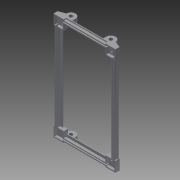
# Autodesk Inventor part: Lid2
Saved by Autodesk Inventor 2015 (Build 190159000, 159)
## iProperties
Created: 2015-03-20
Part Number: Lid2
Material: NylonD2W
Document SubType Name: Modeling
Designer: Akovo_000
Density: 0.93 g/cm^3
Appearance: Nylon 6
Mass: 32.4877 g
Surface Area: 348.455 cm^2
Volume: 34.933 cm^3
Author: Akovo_000
Autodesk Inventor part; units mm, degrees
ref_plane "YZ Plane" through (0, 0, 0) normal (1, 0, 0) x (0, 1, 0)
ref_plane "XZ Plane" through (0, 0, 0) normal (0, 1, 0) x (-1, 0, 0)
ref_plane "Main Work Pane" through (0, 2.75, 7) normal (0, 1, 0) x (-1, 0, 0)
sketch "Panel" plane through (0, 2.75, 7) normal (0, 1, 0) x (-1, 0, 0)
  line L0 (90.0297, -97.7451) -> (-32.1703, -97.7451)
  line L1 (-32.1703, -97.7451) -> (-32.1703, 113.4549)
  line L2 (-32.1703, 113.4549) -> (90.0297, 113.4549)
  line L3 (90.0297, 113.4549) -> (90.0297, -97.7451)
  line L4 (71.9297, 95.3549) -> (88.0297, 95.3549)
  line L5 (88.0297, 95.3549) -> (88.0297, 111.4549)
  line L6 (88.0297, 111.4549) -> (71.9297, 111.4549)
  line L7 (71.9297, 111.4549) -> (71.9297, 95.3549)
  line L8 (69.9297, 113.4549) -> (69.9297, 93.3549)
  line L9 (69.9297, 93.3549) -> (90.0297, 93.3549)
  line L10 (88.0297, -95.7451) -> (71.9297, -95.7451)
  line L11 (71.9297, -95.7451) -> (71.9297, -79.6451)
  line L12 (71.9297, -79.6451) -> (88.0297, -79.6451)
  line L13 (88.0297, -79.6451) -> (88.0297, -95.7451)
  line L14 (90.0297, -77.6451) -> (69.9297, -77.6451)
  line L15 (69.9297, -77.6451) -> (69.9297, -97.7451)
  line L16 (-30.1703, -95.7451) -> (-14.0703, -95.7451)
  line L17 (-14.0703, -95.7451) -> (-14.0703, -79.6451)
  line L18 (-14.0703, -79.6451) -> (-30.1703, -79.6451)
  line L19 (-30.1703, -79.6451) -> (-30.1703, -95.7451)
  line L20 (-12.0703, -97.7451) -> (-12.0703, -77.6451)
  line L21 (-12.0703, -77.6451) -> (-32.1703, -77.6451)
  line L22 (-14.0703, 95.3549) -> (-30.1703, 95.3549)
  line L23 (-30.1703, 95.3549) -> (-30.1703, 111.4549)
  line L24 (-30.1703, 111.4549) -> (-14.0703, 111.4549)
  line L25 (-14.0703, 111.4549) -> (-14.0703, 95.3549)
  line L26 (-12.0703, 113.4549) -> (-12.0703, 93.3549)
  line L27 (-12.0703, 93.3549) -> (-32.1703, 93.3549)
  circle A0 centre (76.9297, 100.3549) radius 2
  circle A1 centre (-19.0703, 100.3549) radius 2
  circle A2 centre (76.9297, -84.6451) radius 2
  circle A3 centre (-19.0703, -84.6451) radius 2
  line L28 (-19.0703, -84.6451) -> (-14.0703, -84.6451) construction
  line L29 (-19.0703, -84.6451) -> (-19.0703, -79.6451) construction
  line L30 (76.9297, -84.6451) -> (71.9297, -84.6451) construction
  line L31 (76.9297, -84.6451) -> (76.9297, -79.6451) construction
  line L32 (76.9297, 100.3549) -> (76.9297, 95.3549) construction
  line L33 (76.9297, 100.3549) -> (71.9297, 100.3549) construction
  line L34 (-19.0703, 100.3549) -> (-14.0703, 100.3549) construction
  line L35 (-19.0703, 100.3549) -> (-19.0703, 95.3549) construction
  line L36 (69.9297, 100.3549) -> (-12.0703, 100.3549)
  line L37 (76.9297, 93.3549) -> (76.9297, -77.6451)
  line L38 (69.9297, -84.6451) -> (-12.0703, -84.6451)
  line L39 (-19.0703, 93.3549) -> (-19.0703, -77.6451)
  dimension "d584" = 2
  dimension "d585" = 2
  dimension "d586" = 2
  dimension "d587" = 2
  dimension "d588" = 16.1
  dimension "d589" = 16.1
  dimension "d592" = 2
  dimension "d593" = 4
  dimension "d597" = 2
  dimension "d648" = 2
  dimension "d661" = 5
  dimension "d670" = 175
  dimension "d671" = 86
  dimension "d682" = 211.2
  dimension "d687" = 122.2
  constraints: 80 end point, 24 point on line, 19 perpendicular, 13 equal length, 10 collinear, 10 parallel, 8 horizontal, 4 centre point, 3 equal radius, 3 vertical
  measures "d584" distance between parallel lines of L2 L6
  measures "d585" distance between parallel lines of L3 L5
  measures "d586" distance between parallel lines of L9 L4
  measures "d587" distance between parallel lines of L7 L8
  measures "d588" distance between parallel lines of L4 L6
  measures "d589" distance between parallel lines of L5 L7
  measures "d592" distance between parallel lines of L1 L19
  measures "d593" diameter of A0
  measures "d597" distance between parallel lines of L0 L10
  measures "d648" distance between parallel lines of L25 L26
  measures "d661" distance of L28.start L29.end
  measures "d670" distance between parallel lines of L12 L4
  measures "d671" distance between parallel lines of L7 L25
  measures "d682" distance between parallel lines of L0 L2
  measures "d687" distance between parallel lines of L1 L3
extrude "FlatPlane" add sketch "Panel" along normal blind 1.5 contours L0 L15 L14 L3 | L0 L20 L38 L15 | L14 L37 L9 L3 | L0 L1 L21 L20 | L9 L8 L2 L3 | L1 L27 L39 L21 | L8 L36 L26 L2 | L1 L2 L26 L27 | L7 L6 L5 L4 | L10 L11 L12 L13 | L19 L18 L17 L16 | L22 L23 L24 L25
sketch "BoardSuport" plane through (0, 2.75, 7) normal (0, -1, 0) x (1, 0, 0)
  line L0 (-90.0297, 113.4549) -> (-69.8297, 113.4549)
  line L1 (-69.8297, 113.4549) -> (-69.8297, 111.4549)
  line L2 (-69.8297, 93.2549) -> (-82.0297, 93.2549)
  line L3 (-90.0297, 93.2549) -> (-90.0297, 113.4549)
  line L4 (32.1703, 113.4549) -> (11.9703, 113.4549)
  line L5 (11.9703, 113.4549) -> (11.9703, 111.4549)
  line L6 (11.9703, 93.2549) -> (24.1703, 93.2549)
  line L7 (32.1703, 93.2549) -> (32.1703, 113.4549)
  line L8 (-90.0297, -97.7451) -> (-69.8297, -97.7451)
  line L9 (-69.8297, -97.7451) -> (-69.8297, -77.5451)
  line L10 (-69.8297, -77.5451) -> (-82.0297, -77.5451)
  line L11 (-90.0297, -77.5451) -> (-90.0297, -97.7451)
  line L12 (32.1703, -97.7451) -> (11.9703, -97.7451)
  line L13 (11.9703, -97.7451) -> (11.9703, -95.7451)
  line L14 (11.9703, -77.5451) -> (24.1703, -77.5451)
  line L15 (32.1703, -77.5451) -> (32.1703, -97.7451)
  line L16 (-90.0297, 93.2549) -> (-88.0297, 93.2549)
  line L17 (-82.0297, 93.2549) -> (-82.0297, -77.5451)
  line L18 (-82.0297, -77.5451) -> (-88.0297, -77.5451)
  line L19 (-90.0297, -77.5451) -> (-90.0297, 93.2549) construction
  line L20 (-69.8297, -97.7451) -> (11.9703, -97.7451) construction
  line L21 (11.9703, -97.7451) -> (11.9703, -89.7451)
  line L22 (11.9703, -89.7451) -> (-69.8297, -89.7451)
  line L23 (-69.8297, -89.7451) -> (-69.8297, -97.7451)
  line L24 (32.1703, -77.5451) -> (30.1703, -77.5451)
  line L25 (24.1703, -77.5451) -> (24.1703, 93.2549)
  line L26 (24.1703, 93.2549) -> (30.1703, 93.2549)
  line L27 (32.1703, 93.2549) -> (32.1703, -77.5451) construction
  line L28 (11.9703, 113.4549) -> (-69.8297, 113.4549) construction
  line L29 (-69.8297, 113.4549) -> (-69.8297, 111.4549)
  line L30 (-69.8297, 105.4549) -> (11.9703, 105.4549)
  line L31 (11.9703, 105.4549) -> (11.9703, 111.4549)
  line L32 (11.9703, -95.7451) -> (-69.8297, -95.7451)
  line L33 (-88.0297, -77.5451) -> (-88.0297, -73.7451)
  line L34 (11.9703, 111.4549) -> (-69.8297, 111.4549)
  line L35 (32.1703, -97.7451) -> (-90.0297, -97.7451) projected
  line L36 (30.1703, -77.5451) -> (30.1703, 93.2549)
  line L37 (-82.0297, -77.5451) -> (-88.0297, -77.5451)
  line L38 (-88.0297, -77.5451) -> (-90.0297, -77.5451)
  line L39 (-69.8297, 105.4549) -> (-69.8297, 93.2549)
  line L40 (-69.8297, 111.4549) -> (-69.8297, 105.4549)
  line L41 (24.1703, 93.2549) -> (30.1703, 93.2549)
  line L42 (30.1703, 93.2549) -> (32.1703, 93.2549)
  line L43 (11.9703, -95.7451) -> (11.9703, -89.7451)
  line L44 (11.9703, -89.7451) -> (11.9703, -77.5451)
  line L45 (30.1703, 93.2549) -> (32.1703, 93.2549)
  line L46 (-88.0297, -73.7451) -> (-88.0297, 93.2549)
  line L47 (-88.0297, 93.2549) -> (-90.0297, 93.2549)
  line L48 (-82.0297, 93.2549) -> (-88.0297, 93.2549)
  line L49 (11.9703, 105.4549) -> (11.9703, 93.2549)
  line L50 (11.9703, 111.4549) -> (11.9703, 105.4549)
  line L51 (30.1703, -77.5451) -> (24.1703, -77.5451)
  line L52 (24.1703, -77.5451) -> (32.1703, -77.5451)
  line L53 (-88.0297, -77.5451) -> (-90.0297, -77.5451)
  line L54 (-88.0297, 93.2549) -> (-82.0297, 93.2549)
  line L55 (11.9703, 111.4549) -> (11.9703, 113.4549)
  line L56 (-69.8297, 111.4549) -> (-69.8297, 105.4549)
  dimension "d617" = 20.2
  dimension "d658" = 2
  dimension "d659" = 6
  dimension "d660" = 20.2
  constraints: 112 end point, 43 parallel, 17 perpendicular, 13 equal length, 10 horizontal, 3 point on line
  measures "d617" distance of L12.end L14.start
  measures "d658" distance between parallel lines of L35 L32
  measures "d659" distance between parallel lines of L32 L22
  measures "d660" distance of L12.end L12.start
extrude "BoardSupport3D" add sketch "BoardSuport" along normal blind 5 contours L0 L1 L40 L39 L2 L48 L16 L3 | L34 L31 L30 L40 | L48 L17 L18 L33 L46 | L5 L4 L7 L42 L26 L6 L49 L31 | L18 L10 L9 L8 L11 L38 | L26 L36 L51 L25 | L22 L21 L32 L9 | L51 L24 L15 L12 L13 L21 L44 L14
sketch "Lens and screwcover" plane through (0, 4.25, 7) normal (0, 1, 0) x (1, 0, 0)
  line L0 (32.1703, 97.7451) -> (11.9703, 97.7451)
  line L1 (11.9703, 97.7451) -> (11.9703, 77.5451)
  line L2 (11.9703, 77.5451) -> (32.1703, 77.5451)
  line L3 (32.1703, 77.5451) -> (32.1703, 97.7451)
  line L4 (-90.0297, 97.7451) -> (-69.8297, 97.7451)
  line L5 (-69.8297, 97.7451) -> (-69.8297, 77.5451)
  line L6 (-69.8297, 77.5451) -> (-90.0297, 77.5451)
  line L7 (-90.0297, 77.5451) -> (-90.0297, 97.7451)
  line L8 (-90.0297, -113.4549) -> (-69.8297, -113.4549)
  line L9 (-69.8297, -113.4549) -> (-69.8297, -93.2549)
  line L10 (-69.8297, -93.2549) -> (-90.0297, -93.2549)
  line L11 (-90.0297, -93.2549) -> (-90.0297, -113.4549)
  line L12 (32.1703, -113.4549) -> (11.9703, -113.4549)
  line L13 (11.9703, -113.4549) -> (11.9703, -93.2549)
  line L14 (11.9703, -93.2549) -> (32.1703, -93.2549)
  line L15 (32.1703, -93.2549) -> (32.1703, -113.4549)
  circle A0 centre (-76.9297, 84.6451) radius 2 projected
  circle A1 centre (-76.9297, 84.6451) radius 2
  circle A2 centre (19.0703, 84.6451) radius 2 projected
  circle A3 centre (19.0703, 84.6451) radius 2
  circle A4 centre (19.0703, -100.3549) radius 2 projected
  circle A5 centre (19.0703, -100.3549) radius 2
  circle A6 centre (-76.9297, -100.3549) radius 2 projected
  circle A7 centre (-76.9297, -100.3549) radius 2
  dimension "d600" = 20.2
  dimension "d601" = 20.2
  constraints: 32 end point, 8 parallel, 6 equal length, 4 centre point, 4 coincident, 4 horizontal, 4 perpendicular, 2 point on line
  measures "d600" distance of L2.end L1.end
  measures "d601" distance of L1.end L0.end
extrude "Extrusion15" add sketch "Lens and screwcover" along normal blind 1.5
sketch "Sketch20" plane through (0, -2.25, 7) normal (0, -1, 0) x (1, 0, 0)
  line L0 (32.1703, 93.2549) -> (32.1703, 113.4549)
  line L1 (32.1703, 113.4549) -> (11.9703, 113.4549)
  line L2 (-69.8297, 93.2549) -> (-90.0297, 93.2549)
  line L3 (-90.0297, 93.2549) -> (-90.0297, 113.4549)
  line L4 (-90.0297, 113.4549) -> (-69.8297, 113.4549)
  line L5 (-69.8297, 113.4549) -> (-69.8297, 93.2549)
  line L6 (32.1703, -97.7451) -> (11.9703, -97.7451)
  line L7 (11.9703, -97.7451) -> (11.9703, -77.5451)
  line L8 (11.9703, -77.5451) -> (32.1703, -77.5451)
  line L9 (32.1703, -77.5451) -> (32.1703, -97.7451)
  line L10 (-69.8297, -77.5451) -> (-90.0297, -77.5451)
  line L11 (-90.0297, -77.5451) -> (-90.0297, -97.7451)
  line L12 (-90.0297, -97.7451) -> (-69.8297, -97.7451)
  line L13 (-69.8297, -97.7451) -> (-69.8297, -77.5451)
  line L14 (13.9703, 95.2549) -> (30.1703, 95.2549)
  line L15 (30.1703, 95.2549) -> (30.1703, 111.4549)
  line L16 (30.1703, 111.4549) -> (13.9703, 111.4549)
  line L17 (13.9703, 111.4549) -> (13.9703, 95.2549)
  line L18 (-71.8297, 95.2549) -> (-88.0297, 95.2549)
  line L19 (-88.0297, 95.2549) -> (-88.0297, 111.4549)
  line L20 (-88.0297, 111.4549) -> (-71.8297, 111.4549)
  line L21 (-71.8297, 111.4549) -> (-71.8297, 95.2549)
  line L22 (-88.0297, -95.7451) -> (-71.8297, -95.7451)
  line L23 (-71.8297, -95.7451) -> (-71.8297, -79.5451)
  line L24 (-71.8297, -79.5451) -> (-88.0297, -79.5451)
  line L25 (-88.0297, -79.5451) -> (-88.0297, -95.7451)
  line L26 (30.1703, -95.7451) -> (13.9703, -95.7451)
  line L27 (13.9703, -95.7451) -> (13.9703, -79.5451)
  line L28 (13.9703, -79.5451) -> (30.1703, -79.5451)
  line L29 (30.1703, -79.5451) -> (30.1703, -95.7451)
  line L30 (-86.0297, 95.2549) -> (-86.0297, -79.5451)
  line L31 (-83.5297, -79.5451) -> (-83.5297, 95.2549)
  line L32 (-71.8297, 109.4549) -> (13.9703, 109.4549)
  line L33 (13.9703, 107.4549) -> (-71.8297, 107.4549)
  line L34 (-71.8297, -93.7451) -> (13.9703, -93.7451)
  line L35 (13.9703, -91.7451) -> (-71.8297, -91.7451)
  line L36 (28.1703, 95.2549) -> (28.1703, -79.5451)
  line L37 (26.1703, -79.5451) -> (26.1703, 95.2549)
  line L38 (11.9703, 93.2549) -> (11.9703, 113.4549)
  line L39 (11.9703, 113.4549) -> (11.9703, 93.2549)
  line L40 (11.9703, 93.2549) -> (32.1703, 93.2549)
  point P0 (0, -7)
  dimension "d620" = 2
  dimension "d621" = 2
  dimension "d622" = 2
  dimension "d623" = 2
  dimension "d626" = 20.2
  dimension "d627" = 20.2
  dimension "d630" = 2
  dimension "d631" = 2.5
  dimension "d632" = 2
  dimension "d633" = 2
  dimension "d634" = 2
  dimension "d635" = 2
  dimension "d636" = 2
  dimension "d637" = 2
  dimension "d652" = 207.2
  dimension "d653" = 174.8
  dimension "d654" = 118.2
  dimension "d668" = 2
  dimension "d669" = 2
  constraints: 82 end point, 21 point on line, 17 equal length, 13 perpendicular, 8 horizontal, 5 collinear, 1 vertical
  measures "d620" distance between parallel lines of L1 L16
  measures "d621" distance between parallel lines of L0 L15
  measures "d622" distance between parallel lines of L6 L26
  measures "d623" distance between parallel lines of L3 L19
  measures "d626" distance between parallel lines of L4 L2
  measures "d627" distance between parallel lines of L3 L5
  measures "d630" distance between parallel lines of L19 L30
  measures "d631" distance between parallel lines of L30 L31
  measures "d632" distance of L20.end L32.start
  measures "d633" distance between parallel lines of L32 L33
  measures "d634" distance of L36.start L14.end
  measures "d635" distance between parallel lines of L37 L36
  measures "d636" distance between parallel lines of L35 L34
  measures "d637" distance from line of L22.end L34
  measures "d652" distance between parallel lines of L16 L26
  measures "d653" distance between parallel lines of L14 L28
  measures "d654" distance between parallel lines of L15 L19
  measures "d668" distance between parallel lines of L40 L14
  measures "d669" distance between parallel lines of L38 L17
extrude "Extrusion17" cut sketch "Sketch20" against normal blind 5 contours L40 L37 L14 L36 | L36 L8 L37 L40 | L14 L17 L16 L15 | L36 L28 L37 L8 | L38 L33 L5 L32 | L32 L17 L33 L38 | L28 L29 L26 L27 | L5 L33 L21 L32 | L21 L18 L19 L20 | L35 L27 L34 L7 | L7 L34 L13 L35 | L13 L34 L23 L35 | L31 L10 L30 L2 | L2 L30 L18 L31 | L23 L22 L25 L24 | L31 L24 L30 L10
sketch "Sketch22" plane through (-69.8297, 2.75, 120.4549) normal (0, 0, 1) x (1, 0, 0)
  line L0 (-20.2, 1.5) -> (-20.2, 7.6756) construction
  line L1 (102, 7.6756) -> (102, 1.5) construction
  line L2 (-20.2, 1.5) -> (102, 1.5)
  line L3 (1.4205, 7.6756) -> (80.3795, 7.6756) construction
  circle A0 centre (1.4205, 7.6756) radius 3.5
  circle A1 centre (80.3795, 7.6756) radius 3.5
  line L4 (1.4205, 7.6756) -> (-20.2, 7.6756) construction
  line L5 (80.3795, 7.6756) -> (102, 7.6756) construction
  arc A2 (10.4205, 7.6756) -> (-7.5795, 7.6756) centre (1.4205, 7.6756) ccw
  arc A3 (89.3795, 7.6756) -> (71.3795, 7.6756) centre (80.3795, 7.6756) ccw
  line L6 (10.4205, 7.6756) -> (10.4205, 1.5)
  line L7 (71.3795, 7.6756) -> (71.3795, 1.5)
  line L8 (0, 1.5) -> (81.8, 1.5) projected
  line L9 (-20.2, 3) -> (-20.2, -5) projected
  line L10 (102, 3) -> (102, -5) projected
  line L11 (89.3795, 7.6756) -> (89.3795, 3)
  line L12 (-20.2, 3) -> (-7.5795, 7.6756)
  line L13 (89.3795, 7.6756) -> (102, 3)
  line L14 (-20.2, 1.5) -> (10.4205, 1.5)
  line L15 (-20.2, 3) -> (-20.2, 1.5)
  line L16 (0, 3) -> (-20.2, 3) projected
  line L17 (102, 3) -> (102, 1.5)
  line L18 (102, 1.5) -> (71.3795, 1.5)
  point P0 (171.8029, 0.2464)
  point P1 (191, 3)
  dimension "d673" = 7
  dimension "d679" = 9
  constraints: 30 end point, 6 collinear, 6 perpendicular, 5 point on line, 4 centre point, 4 coincident, 4 point on circle, 3 vertical, 2 equal radius, 2 tangent, 1 horizontal
  measures "d673" diameter of A0
  measures "d679" radius of A2
extrude "Extrusion18" add sketch "Sketch22" against normal blind 9
sketch "Sketch23" plane through (11.9703, 2.75, -90.7451) normal (0, 0, -1) x (-1, 0, 0)
  line L0 (-20.2, 1.5) -> (-20.2, 7.6756) construction
  line L1 (102, 7.6756) -> (102, 1.5) construction
  line L2 (-20.2, 1.5) -> (102, 1.5)
  line L3 (1.4205, 7.6756) -> (80.3795, 7.6756) construction
  circle A0 centre (1.4205, 7.6756) radius 3.5
  circle A1 centre (80.3795, 7.6756) radius 3.5
  line L4 (1.4205, 7.6756) -> (-20.2, 7.6756) construction
  line L5 (80.3795, 7.6756) -> (102, 7.6756) construction
  arc A2 (10.4205, 7.6756) -> (-7.5795, 7.6756) centre (1.4205, 7.6756) ccw
  arc A3 (89.3795, 7.6756) -> (71.3795, 7.6756) centre (80.3795, 7.6756) ccw
  line L6 (10.4205, 7.6756) -> (10.4205, 1.5)
  line L7 (71.3795, 7.6756) -> (71.3795, 1.5)
  line L8 (0, 1.5) -> (81.8, 1.5)
  line L9 (-20.2, 3) -> (-20.2, -5)
  line L10 (102, 3) -> (102, -5)
  line L11 (89.3795, 7.6756) -> (89.3795, 3)
  line L12 (-20.2, 3) -> (-7.5795, 7.6756)
  line L13 (89.3795, 7.6756) -> (102, 3)
  line L14 (-20.2, 1.5) -> (10.4205, 1.5)
  line L15 (-20.2, 3) -> (-20.2, 1.5)
  line L16 (0, 3) -> (-20.2, 3)
  line L17 (102, 3) -> (102, 1.5)
  line L18 (102, 1.5) -> (71.3795, 1.5)
  point P0 (11.9703, -2.75)
  point P1 (171.8029, 0.2464)
  point P2 (191, 3)
  dimension "d683" = 7
  dimension "d684" = 9
  constraints: 38 end point, 6 collinear, 6 perpendicular, 5 point on line, 4 centre point, 4 coincident, 4 point on circle, 3 vertical, 2 equal radius, 2 tangent, 1 horizontal
  measures "d683" diameter of A0
  measures "d684" radius of A2
extrude "Extrusion19" add sketch "Sketch23" against normal blind 9
body "Solid3"
